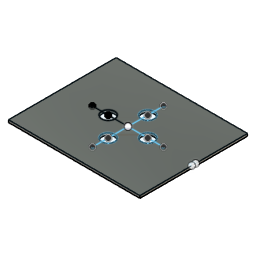
simon (Autodesk Fusion 360 design; units mm, degrees)
Autodesk Fusion 360 part; units mm, degrees
box "BoxPrimitive1" add length 136 width 166 height 3 placed x (0, -1, 0) y (1, 0, 0) z (0, 0, 1) at (-30, 40, 0)
move_body "Move1" bodies 1 to x (1, 0, 0) y (0, 1, 0) z (0, 0, 1) at (-59.3373, 23.0424, 23.0424)
move_body "Move2" bodies 1 to x (1, 0, 0) y (0, 1, 0) z (0, 0, 1) at (6.3373, 4.9576, -26.0424)
move_body "Move3" bodies 1 to x (1, 0, 0) y (0, 1, 0) z (0, 0, 1) at (0, 0, 3)
sketch "Sketch6" plane through (0, 0, 3) normal (0, 0, 1) x (-1, 0, 0)
  line L0 (83, 68) -> (-83, 68)
  line L1 (-83, 68) -> (-83, -68)
  line L2 (-83, -68) -> (83, -68)
  line L3 (83, -68) -> (83, 68)
  line L4 (0, 0) -> (25, 0)
  line L5 (25, 0) -> (45, 0)
  circle A0 centre (25, 0) radius 8.25
  line L6 (44, -1.5) -> (46, -1.5)
  line L7 (46, -1.5) -> (46, 1.5)
  line L8 (46, 1.5) -> (44, 1.5)
  line L9 (44, 1.5) -> (44, -1.5)
  line L10 (44, -1.5) -> (46, 1.5) construction
  line L11 (46, -1.5) -> (44, 1.5) construction
  line L12 (0, 0) -> (0, -25)
  line L13 (1.5, -44) -> (-1.5, -44)
  line L14 (0, -25) -> (0, -45)
  line L15 (-1.5, -46) -> (1.5, -44) construction
  circle A1 centre (0, -25) radius 8.25
  line L16 (-1.5, -44) -> (-1.5, -46)
  line L17 (1.5, -46) -> (1.5, -44)
  line L18 (-1.5, -44) -> (1.5, -46) construction
  line L19 (-1.5, -46) -> (1.5, -46)
  line L20 (-44, 1.5) -> (-46, -1.5) construction
  line L21 (0, 0) -> (-25, 0)
  line L22 (-1.5, 44) -> (1.5, 44)
  line L23 (0, 25) -> (0, 45)
  line L24 (-44, 1.5) -> (-46, 1.5)
  circle A2 centre (0, 25) radius 8.25
  line L25 (-1.5, 46) -> (-1.5, 44)
  line L26 (-25, 0) -> (-45, 0)
  line L27 (1.5, 44) -> (1.5, 46)
  line L28 (-46, 1.5) -> (-44, -1.5) construction
  line L29 (1.5, 46) -> (-1.5, 46)
  line L30 (-46, 1.5) -> (-46, -1.5)
  line L31 (1.5, 46) -> (-1.5, 44) construction
  line L32 (-44, -1.5) -> (-44, 1.5)
  circle A3 centre (-25, 0) radius 8.25
  line L33 (-46, -1.5) -> (-44, -1.5)
  line L34 (0, 0) -> (0, 25)
  line L35 (1.5, 44) -> (-1.5, 46) construction
  line L36 (-80.4869, -2.4905) -> (-83, -2.4905)
  line L37 (-83, 2.5095) -> (-80.4869, 2.5095)
  line L38 (-80.4869, 2.5095) -> (-80.4869, -2.4905)
  point P0 (45, 0)
  point P1 (0, -45)
  point P2 (-45, 0)
  point P3 (0, 45)
  dimension "d26" = 25
  dimension "d27" = 20
  dimension "d28" = 16.5
  dimension "d29" = 2
  dimension "d30" = 3
  dimension "d31" = 25
  dimension "d32" = 20
  dimension "d33" = 16.5
  dimension "d34" = 2
  dimension "d35" = 3
  dimension "d36" = 25
  dimension "d37" = 20
  dimension "d38" = 16.5
  dimension "d39" = 2
  dimension "d40" = 3
  dimension "d41" = 25
  dimension "d42" = 20
  dimension "d43" = 16.5
  dimension "d44" = 2
  dimension "d45" = 3
  dimension "d48" = 5
  constraint coincident L4.start L12.start
  constraint horizontal L4
  constraint parallel L4 L5
  constraint coincident L4.end L5.start
  constraint horizontal L6
  constraint perpendicular L6 L7
  constraint parallel L6 L8
  constraint parallel L7 L9
  constraint coincident L10 P0
  constraint coincident L11 P0
  constraint coincident P0 L5.end
  constraint parallel L12 L14
  constraint coincident L12.end L14.start
  constraint perpendicular L16 L19
  constraint parallel L16 L17
  constraint parallel L13 L19
  constraint coincident P1 L18
  constraint coincident P1 L15
  constraint coincident P1 L14.end
  constraint parallel L21 L26
  constraint coincident L21.end L26.start
  constraint perpendicular L24 L30
  constraint parallel L24 L33
  constraint parallel L30 L32
  constraint coincident P2 L20
  constraint coincident P2 L28
  constraint coincident P2 L26.end
  constraint parallel L23 L34
  constraint coincident L23.start A2.centre
  constraint perpendicular L27 L29
  constraint parallel L25 L27
  constraint parallel L22 L29
  constraint coincident P3 L35
  constraint coincident P3 L31
  constraint coincident P3 L23.end
  constraint horizontal L36
  constraint horizontal L37
  constraint vertical L38
  measures "d26" distance of L4.start L4.end
  measures "d27" distance of L4.end P0
  measures "d28" diameter of A0
  measures "d29" distance of L7.end L8.end
  measures "d30" distance of L6.end L7.end
  measures "d31" distance of L4.start L12.end
  measures "d32" distance of L12.end P1
  measures "d33" diameter of A1
  measures "d34" distance of L17.start L13.start
  measures "d35" distance of L15.start L17.start
  measures "d36" distance of L4.start L21.end
  measures "d37" distance of L21.end P2
  measures "d38" diameter of A3
  measures "d39" distance of L20.end L28.end
  measures "d40" distance of L24.end L20.end
  measures "d41" distance of L4.start L23.start
  measures "d42" distance of P3 L23.start
  measures "d43" diameter of A2
  measures "d44" distance of L22.start L25.start
  measures "d45" distance of L27.end L25.start
  measures "d48" distance of L36.start L37.end
extrude "Extrude2" cut sketch "Sketch6" against normal blind 5 contours L4 L5 A0 | L4 L5 A0 | L6 L7 L8 L9 | L12 L14 A1 | L12 L14 A1 | L13 L16 L17 L19 | L21 L26 A3 | L21 L26 A3 | L22 L25 L27 L29 | L23 A2 L34 | L23 A2 L34 | L24 L30 L32 L33
